Placeholder_Pin_MountFitTesting (Autodesk Fusion 360 design; units mm, degrees)
part number: 2026-09-18-15-20-36-861
Autodesk Fusion 360 part; units mm, degrees
sketch "Sketch1" plane through (0, 0, 0) normal (0, 0, 1) x (1, 0, 0)
  circle A0 centre (0, 0) radius 1.15
  dimension "d1" = 2.3
  constraint coincident A0.centre origin
  measures "d1" diameter of A0
extrude "Extrude1" add sketch "Sketch1" along normal blind 5
